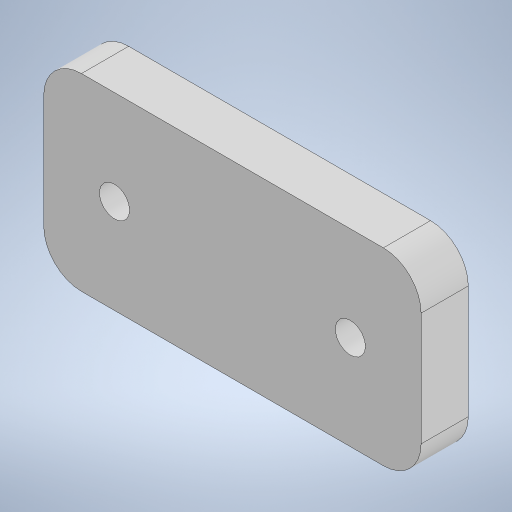
# Autodesk Inventor part: Spacer
Saved by Autodesk Inventor 2023.1 (Build 271208000, 208)
## iProperties
Created: 2022-11-21
Part Number: Spacer
Material: Generic
Document SubType Name: Modeling
Designer: nicol
Density: 1 g/cm^3
Appearance: Default
Author: nicol
Autodesk Inventor part; units mm, degrees
ref_plane "YZ Plane" through (0, 0, 0) normal (1, 0, 0) x (0, 1, 0)
ref_plane "XZ Plane" through (0, 0, 0) normal (0, 1, 0) x (-1, 0, 0)
ref_plane "XY Plane" through (0, 0, 0) normal (0, 0, 1) x (1, 0, 0)
sketch "Sketch1" plane through (0, 0, 0) normal (0, 0, 1) x (1, 0, 0)
  line L0 (0, 0) -> (40, 0)
  line L1 (40, 0) -> (40, 20)
  line L2 (40, 20) -> (0, 20)
  line L3 (0, 20) -> (0, 0)
  point P0 (7.5, 10)
  point P1 (32.5, 10)
  point P2 (40, 10)
  dimension "d0" = 20
  dimension "d1" = 7.5
  dimension "d2" = 7.5
  dimension "d3" = 25
  constraints: 8 end point, 2 horizontal alignment, 2 parallel, 1 horizontal, 1 midpoint, 1 perpendicular
  measures "d0" distance of L1.end L0.end
  measures "d1" distance from line of L1 point (32.5, 10)
  measures "d2" distance from line of L3 point (7.5, 10)
  measures "d3" distance of point (32.5, 10) point (7.5, 10)
extrude "Extrusion1" add sketch "Sketch1" against normal blind 5
hole "Hole1" at (7.5, 10, 0) at (32.5, 10, 0) direction (0, 0, -1) diameter 3.2 depth 25.4 tip angle 118
fillet "Fillet1" radius 4 4 edges at (40, 20, -2.5) (40, 0, -2.5) (0, 0, -2.5) (0, 20, -2.5)
body "Solid1"
